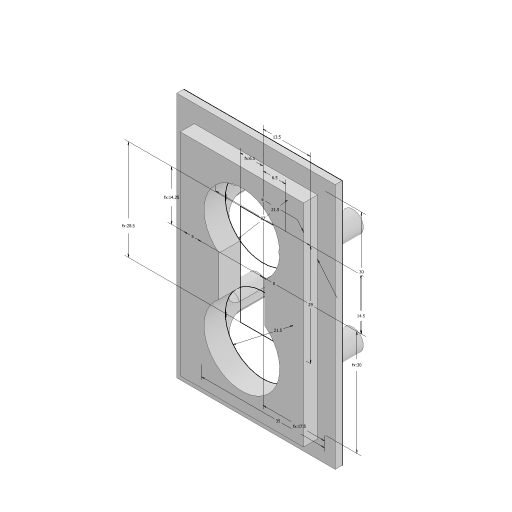
# Autodesk Inventor part: lidar_lite_v3_lidar_mount
Saved by Autodesk Inventor 2023 (Build 270158000, 158)
## iProperties
Created: 2022-05-19
Part Number: lidar_lite_v3_lidar_mount
Material: Generic
Document SubType Name: Modeling
Designer: Thomas
Density: 1 g/cm^3
Appearance: Default
Author: Thomas
Autodesk Inventor part; units mm, degrees
ref_plane "YZ Plane" through (0, 0, 0) normal (1, 0, 0) x (0, 1, 0)
ref_plane "XZ Plane" through (0, 0, 0) normal (0, 1, 0) x (-1, 0, 0)
ref_plane "XY Plane" through (0, 0, 0) normal (0, 0, 1) x (1, 0, 0)
sketch "Sketch1" plane through (0, 0, 0) normal (0, 0, 1) x (1, 0, 0)
  circle A0 centre (0, 14.25) radius 10.75
  circle A1 centre (0, -14.25) radius 10.75
  line L0 (0, 14.25) -> (0, -14.25) construction
  line L1 (-17.5, 30) -> (17.5, 30)
  line L2 (17.5, 30) -> (17.5, -30)
  line L3 (17.5, -30) -> (-17.5, -30)
  line L4 (-17.5, -30) -> (-17.5, 30)
  line L5 (-22.5, 35) -> (22.5, 35)
  line L6 (22.5, 35) -> (22.5, -35)
  line L7 (22.5, -35) -> (-22.5, -35)
  line L8 (-22.5, -35) -> (-22.5, 35)
  line L9 (-6.5, 14.25) -> (6.5, 14.25)
  line L10 (6.5, 14.25) -> (6.5, -14.25)
  line L11 (6.5, -14.25) -> (-6.5, -14.25)
  line L12 (-6.5, -14.25) -> (-6.5, 14.25)
  circle A2 centre (13.5, 14.5) radius 3
  circle A3 centre (-13.5, 14.5) radius 3
  circle A4 centre (13.5, -14.5) radius 3
  circle A5 centre (-13.5, -14.5) radius 3
  point P0 (0, 0)
  point P1 (-5.8896, 0)
  point P2 (5.8896, 0)
  point P3 (0, 0)
  point P4 (6.5, 5.6877)
  point P5 (10.7151, 13.3845)
  point P6 (10.6757, 15.5116)
  point P7 (-6.5, 5.6877)
  point P8 (-6.5, -5.6877)
  point P9 (6.5, -5.6877)
  point P10 (10.7151, -13.3845)
  point P11 (10.6757, -15.5116)
  point P12 (-10.6757, -15.5116)
  point P13 (-10.7151, -13.3845)
  point P14 (-10.7151, 13.3845)
  point P15 (-10.6757, 15.5116)
  dimension "d0" = 21.5
  dimension "d1" = 21.5
  dimension "d2" = 28.5
  dimension "d3" = 14.25
  dimension "d6" = 0
  dimension "d13" = 35
  dimension "d14" = 17.5
  dimension "d15" = 30
  dimension "d16" = 30
  dimension "d17" = 5
  dimension "d22" = 6.5
  dimension "d23" = 6.5
  dimension "d24" = 6
  dimension "d25" = 14.5
  dimension "d26" = 13.5
  dimension "d36" = 27
  dimension "d39" = 29
  constraints: 26 end point, 6 centre point, 6 parallel, 3 horizontal, 3 midpoint, 3 perpendicular, 2 vertical, 9 other
  measures "d0" diameter of A0
  measures "d1" diameter of A1
  measures "d2" distance of L0.start L0.end
  measures "d3" distance of point (0, 0) L0.start
  measures "d6" distance from line of point (0, 0) L0
  measures "d13" distance of L2.end L3.end
  measures "d14" distance from line of point (0, 0) L2
  measures "d15" distance from line of point (0, 0) L1
  measures "d16" distance from line of point (0, 0) L3
  measures "d17" distance between parallel lines of L4 L8
  measures "d22" distance from line of point (0, 0) L10
  measures "d23" distance from line of point (0, 0) L12
  measures "d24" diameter of A2
  measures "d25" vertical distance of point (0, 0) A2.centre
  measures "d26" horizontal distance of point (0, 0) A2.centre
  measures "d36" distance of A2.centre A3.centre
  measures "d39" distance of A2.centre A4.centre
extrude "Extrusion1" add sketch "Sketch1" along normal blind 2 contours A0 A2 | A0 A2 | A2 A0 L10 L9 L12 A3 | A3 A0 | A0 A3 | L10 A1 L12 A0 | A0 L12 L9 L10 | L10 L11 L12 A1 | A1 A4 A5 L12 L11 L10 | A4 A1 | A1 A4 | A5 A1 | A1 A5 | L1 L2 L3 L4 | L5 L6 L7 L8
extrude "Extrusion2" add sketch "Sketch1" along normal blind 6 contours A0 A2 | A0 A2 | A2 A0 L10 L9 L12 A3 | A3 A0 | A0 A3 | L10 A1 L12 A0 | A0 L12 L9 L10 | L10 L11 L12 A1 | A1 A4 A5 L12 L11 L10 | A4 A1 | A1 A4 | A5 A1 | A1 A5 | L1 L2 L3 L4
extrude "Extrusion3" cut sketch "Sketch1" along normal through all contours A2 A0 L10 L9 L12 A3 | A3 A0 | L10 A1 L12 A0 | A0 L12 L9 L10 | L10 L11 L12 A1 | A1 A4 A5 L12 L11 L10 | A1 A4 | A5 A1 picked at (-10.6615, 14.466) picked at (10.5983, -14.3799) picked at (-10.6615, -14.466)
extrude "Extrusion4" add sketch "Sketch1" against normal blind 12 contours A0 A2 | A0 A3 | A4 A1 | A1 A5 picked at (14.5563, 14.6477) picked at (-14.568, 14.4014) picked at (14.5563, -14.6477) picked at (-14.568, -14.4014)
sketch "Sketch2" plane through (0, 0, -12) normal (0, 0, -1) x (-1, 0, 0)
  arc A0 (-10.6757, 15.5116) -> (-10.7151, 13.3845) centre (0, 14.25) ccw projected
  arc A1 (-10.6757, 15.5116) -> (-10.7151, 13.3845) centre (-13.5, 14.5) ccw projected
  circle A2 centre (-13.5, 14.5) radius 2.05
  arc A3 (-10.7151, -13.3845) -> (-10.6757, -15.5116) centre (0, -14.25) ccw projected
  arc A4 (-10.7151, -13.3845) -> (-10.6757, -15.5116) centre (-13.5, -14.5) ccw projected
  arc A5 (10.6757, -15.5116) -> (10.7151, -13.3845) centre (0, -14.25) ccw projected
  arc A6 (10.6757, -15.5116) -> (10.7151, -13.3845) centre (13.5, -14.5) ccw projected
  arc A7 (10.7151, 13.3845) -> (10.6757, 15.5116) centre (0, 14.25) ccw projected
  arc A8 (10.7151, 13.3845) -> (10.6757, 15.5116) centre (13.5, 14.5) ccw projected
  circle A9 centre (13.5, 14.5) radius 2.05
  circle A10 centre (13.5, -14.5) radius 2.05
  circle A11 centre (-13.5, -14.5) radius 2.05
  point P0 (0, 0)
  dimension "d31" = 4.1
  dimension "d42" = 4.1
  dimension "d43" = 4.1
  dimension "d44" = 4.1
  constraints: 4 centre point, 4 coincident
  measures "d31" diameter of A2
  measures "d42" diameter of A9
  measures "d43" diameter of A10
  measures "d44" diameter of A11
extrude "Extrusion5" cut sketch "Sketch2" against normal blind 5 draft -3 contours A2 | A9 | A10 | A11
fillet "Fillet1" radius 4 4 edges at (16.4995, 14.5555, 0) (-16.4995, 14.5555, 0) (-16.4995, -14.5555, 0) (16.4995, -14.5555, 0)
equation "\"d3\" = 0.5 * d2"
equation "\"d14\" = 0.5 * d13"
equation "\"d16\" = d15"
equation "\"d23\" = d22"
body "Solid1"
